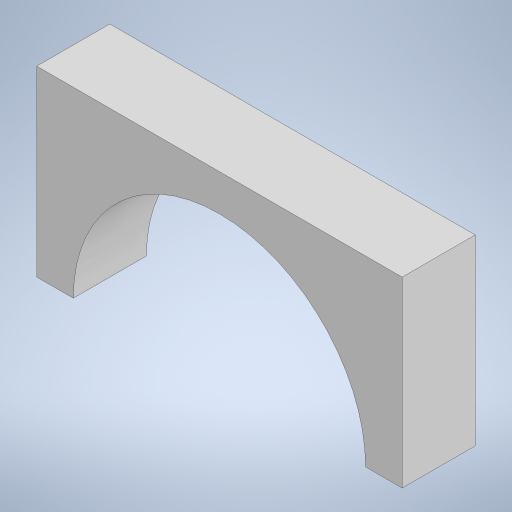
# Autodesk Inventor part: fixation_pipe_v01
Saved by Autodesk Inventor 2023 (Build 270158000, 158)
## iProperties
Created: 2021-04-13
Part Number: fixation_pipe_v01
Material: Generic
Document SubType Name: Modeling
Designer: KAMPFF-LAB-BEHAVIOR
Density: 1 g/cm^3
Appearance: Default
Author: KAMPFF-LAB-BEHAVIOR
Autodesk Inventor part; units mm, degrees
ref_plane "YZ Plane" through (0, 0, 0) normal (1, 0, 0) x (0, 1, 0)
ref_plane "XZ Plane" through (0, 0, 0) normal (0, 1, 0) x (-1, 0, 0)
ref_plane "XY Plane" through (0, 0, 0) normal (0, 0, 1) x (1, 0, 0)
sketch "Sketch13" plane through (0, 0, 0) normal (0, 0, 1) x (1, 0, 0)
  line L0 (-50, 50) -> (50, 50)
  line L1 (50, 50) -> (50, 0)
  line L2 (50, 0) -> (-50, 0)
  line L3 (-50, 0) -> (-50, 50)
  line L4 (-50, 50) -> (50, 0) construction
  line L5 (50, 50) -> (-50, 0) construction
  point P0 (0, 0)
  point P1 (0, 25)
  dimension "d42" = 100
  dimension "d43" = 50
  constraints: 12 end point, 2 midpoint, 2 parallel, 1 horizontal, 1 perpendicular
  measures "d42" distance of L1.end L2.end
  measures "d43" distance of L0.end L1.end
extrude "Extrusion11" add sketch "Sketch13" along normal blind 20
sketch "Sketch14" plane through (0, 0, 20) normal (0, 0, 1) x (1, 0, 0)
  circle A0 centre (0, 0) radius 40
  dimension "d46" = 80
  constraints: 1 centre point, 1 coincident
  measures "d46" diameter of A0
extrude "Extrusion12" cut sketch "Sketch14" against normal blind 20
body "Solid3"
